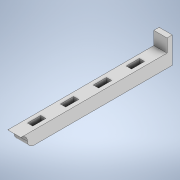
# Autodesk Inventor part: держак середины пушки
Saved by Autodesk Inventor 2020.1 (Build 241239000, 239)
## iProperties
Created: 2022-03-19
Part Number: держак середины пушки
Material: Типовые
Document SubType Name: Modeling
Designer: User
Density: 1 g/cm^3
Appearance: По умолчанию
Author: User
Autodesk Inventor part; units mm, degrees
ref_plane "YZ Plane" through (0, 0, 0) normal (1, 0, 0) x (0, 1, 0)
ref_plane "XZ Plane" through (0, 0, 0) normal (0, 1, 0) x (-1, 0, 0)
ref_plane "XY Plane" through (0, 0, 0) normal (0, 0, 1) x (1, 0, 0)
sketch "Эскиз1" plane through (0, 0, 0) normal (1, 0, 0) x (0, 1, 0)
  line L0 (0, 0) -> (10, 0)
  line L1 (10, 0) -> (10, -110)
  line L2 (10, -110) -> (0, -110)
  line L3 (0, -110) -> (0, 0)
  line L4 (10, -110) -> (20, -110)
  line L5 (20, -110) -> (20, -106)
  line L6 (20, -106) -> (10, -106)
  line L7 (10, -106) -> (10, -110)
  dimension "d0" = 110
  dimension "d1" = 10
  dimension "d2" = 4
  dimension "d3" = 10
  constraints: 16 end point, 4 parallel, 2 horizontal, 2 perpendicular
  measures "d0" distance of L0.end L1.end
  measures "d1" distance of L0.start L0.end
  measures "d2" distance of L4.end L5.end
  measures "d3" distance of L5.end L6.end
extrude "Выдавливание1" add sketch "Эскиз1" along normal blind 10
sketch "Эскиз2" plane through (0, 10, 0) normal (0, 1, 0) x (1, 0, 0)
  line L0 (0, 106) -> (10, 106) projected
  line L1 (5, 106) -> (5, 0)
  line L2 (0, 0) -> (10, 0) projected
  line L3 (7, 82) -> (3, 82)
  line L4 (3, 82) -> (3, 92)
  line L5 (3, 92) -> (7, 92)
  line L6 (7, 92) -> (7, 82)
  line L7 (7, 57) -> (3, 57)
  line L8 (3, 57) -> (3, 67)
  line L9 (3, 67) -> (7, 67)
  line L10 (7, 67) -> (7, 57)
  line L11 (7, 32) -> (3, 32)
  line L12 (3, 32) -> (3, 42)
  line L13 (3, 42) -> (7, 42)
  line L14 (7, 42) -> (7, 32)
  line L15 (7, 7) -> (3, 7)
  line L16 (3, 7) -> (3, 17)
  line L17 (3, 17) -> (7, 17)
  line L18 (7, 17) -> (7, 7)
  dimension "d6" = 10
  dimension "d7" = 10
  dimension "d8" = 10
  dimension "d9" = 10
  dimension "d10" = 4
  dimension "d11" = 4
  dimension "d12" = 4
  dimension "d13" = 14
  dimension "d14" = 15
  dimension "d15" = 15
  dimension "d16" = 15
  constraints: 34 end point, 8 parallel, 4 horizontal, 4 perpendicular, 2 midpoint, 1 point on line, 4 other
  measures "d6" distance of L5.end L3.start
  measures "d7" distance of L9.end L7.start
  measures "d8" distance of L13.end L11.start
  measures "d9" distance of L17.end L15.start
  measures "d10" distance of L4.end L5.end
  measures "d11" distance of L8.end L9.end
  measures "d12" distance of L16.end L17.end
  measures "d13" distance from line of L0 L5.end
  measures "d14" distance of L9.end L3.start
  measures "d15" distance of L7.start L13.end
  measures "d16" distance of L11.start L17.end
extrude "Выдавливание2" cut sketch "Эскиз2" against normal blind 4
sketch "Эскиз3" plane through (10, 0, 0) normal (1, 0, 0) x (0, 0, -1)
  line L0 (106, 10) -> (0, 10) projected
  line L1 (0, 10) -> (-10, 10)
  line L2 (-10, 10) -> (-10, 0)
  line L3 (-10, 0) -> (0, 0)
  line L4 (0, 0) -> (0, 10)
  circle A0 centre (-5, 5) radius 5
  point P0 (-5, 10)
  point P1 (0, 5)
  dimension "d19" = 10
  constraints: 8 end point, 2 parallel, 1 centre point, 1 horizontal, 1 perpendicular
  measures "d19" distance of L3.end L2.end
extrude "Выдавливание3" add sketch "Эскиз3" against normal blind 10 contours L4 A0 L1
fillet "Сопряжение1" radius 5 1 edges at (5, 0, 0)
